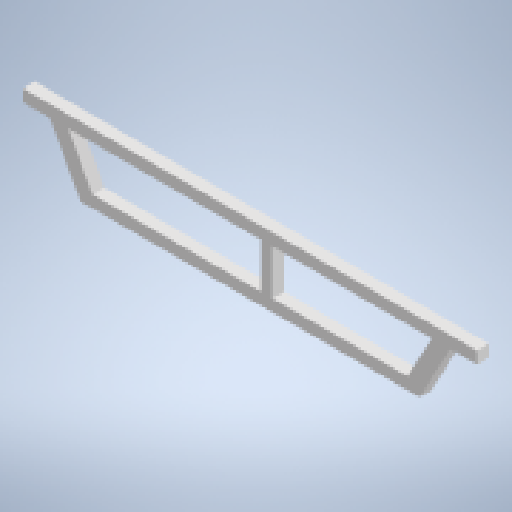
# Autodesk Inventor part: DOF7
Saved by Autodesk Inventor 2024 (Build 280153000, 153)
## iProperties
Created: 2024-10-16
Part Number: DOF7
Material: 一般
Document SubType Name: Modeling
Designer: jerry
Density: 1 g/cm^3
Appearance: 預設
Author: jerry
Autodesk Inventor part; units mm, degrees
ref_plane "YZ Plane" through (0, 0, 0) normal (1, 0, 0) x (0, 1, 0)
ref_plane "XZ Plane" through (0, 0, 0) normal (0, 1, 0) x (-1, 0, 0)
ref_plane "XY Plane" through (0, 0, 0) normal (0, 0, 1) x (1, 0, 0)
sketch "草圖1" plane through (0, 0, 0) normal (0, 0, 1) x (1, 0, 0)
  line L0 (0, 0) -> (115, 0)
  line L1 (0, 0) -> (-450, 0)
  line L2 (-167.5, 95) -> (135, 95)
  line L3 (-167.5, 95) -> (-470, 95)
  line L4 (-167.5, 20) -> (95, 20)
  line L5 (-167.5, 20) -> (-430, 20)
  line L6 (-430, 20) -> (-470, 95)
  line L7 (95, 20) -> (135, 95)
  line L8 (115, 0) -> (165.6667, 95)
  line L9 (165.6667, 95) -> (210.6667, 95)
  line L10 (210.6667, 95) -> (210.6667, 115)
  line L11 (210.6667, 115) -> (-559.3333, 115)
  line L12 (-450, 0) -> (-500.6667, 95)
  line L13 (-500.6667, 95) -> (-545.6667, 95)
  line L14 (-545.6667, 95) -> (-545.6667, 115)
  line L15 (-130, 20) -> (-130, 95)
  line L16 (-130, 20) -> (-150, 20)
  line L17 (-150, 20) -> (-150, 95)
  dimension "d0" = 115
  dimension "d2" = 450
  dimension "d5" = 302.5
  dimension "d6" = 302.5
  dimension "d8" = 262.5
  dimension "d9" = 262.5
  dimension "d10" = 45
  dimension "d11" = 20
  dimension "d13" = 770
  dimension "d14" = 45
  dimension "d16" = 20
  constraints: 36 end point, 6 point on line, 5 horizontal, 5 parallel, 4 perpendicular, 1 coincident
  measures "d0" distance of L0.start L0.end
  measures "d2" distance of L1.start L1.end
  measures "d5" distance of L2.start L2.end
  measures "d6" distance of L2.start L3.end
  measures "d8" distance of L4.start L4.end
  measures "d9" distance of L4.start L5.end
  measures "d10" distance of L8.end L9.end
  measures "d11" distance of L9.end L10.end
  measures "d13" distance of L10.end L11.end
  measures "d14" distance of L12.end L13.end
  measures "d16" distance of L15.start L16.end
extrude "擠出1" add sketch "草圖1" along normal blind 20 contours L1 L12 L13 L14 L11 L10 L9 L8 L0 | L2 L15 L4 L17
sketch "草圖2" plane through (-545.6667, 115, 0) normal (0, 1, 0) x (1, 0, 0)
  line L0 (756.3333, 0) -> (756.3333, -20) projected
  circle A0 centre (723.8333, -10) radius 5
  line L1 (0, 0) -> (0, -20) projected
  circle A1 centre (32.5, -10) radius 5
  point P0 (545.6667, 0)
  dimension "d21" = 10
  dimension "d23" = 10
  constraints: 2 centre point
  measures "d21" diameter of A0
  measures "d23" diameter of A1
extrude "擠出2" add sketch "草圖2" along normal blind 20
sketch "草圖3" plane through (-513.1667, 135, 10) normal (0, 1, 0) x (1, 0, 0)
  circle A0 centre (0, 0) radius 5 projected
  circle A1 centre (0, 0) radius 17.5
  point P0 (513.1667, 10)
  dimension "d26" = 35
  constraints: 1 centre point, 1 coincident
  measures "d26" diameter of A1
extrude "擠出3" add sketch "草圖3" along normal blind 10 contours A0 | A1
sketch "草圖4" plane through (178.1667, 135, 10) normal (0, 1, 0) x (1, 0, 0)
  circle A0 centre (0, 0) radius 17.5
  point P0 (-178.1667, 10)
  dimension "d29" = 35
  constraints: 1 centre point
  measures "d29" diameter of A0
extrude "擠出4" add sketch "草圖4" along normal blind 10
